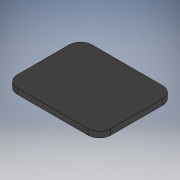
# Autodesk Inventor part: PODUSZKA PODSTAWY
Saved by Autodesk Inventor 2017 SP1 (Build 210196100, 196)
## iProperties
Created: 2020-12-24
Part Number: PODUSZKA PODSTAWY
Material: Kauczuk, silikon
Document SubType Name: Modeling
Designer: Napoleon
Mass: 0.902038 g
Surface Area: 10.8795 cm^2
Volume: 0.72163 cm^3
Density: 1.25 g/cm^3
Appearance: Kauczuk — czarny
Author: Napoleon
Autodesk Inventor part; units mm, degrees
ref_plane "YZ Plane" through (0, 0, 0) normal (1, 0, 0) x (0, 1, 0)
ref_plane "XZ Plane" through (0, 0, 0) normal (0, 1, 0) x (-1, 0, 0)
ref_plane "XY Plane" through (0, 0, 0) normal (0, 0, 1) x (1, 0, 0)
sketch "Szkic1" plane through (0, 0, 0) normal (0, 0, 1) x (1, 0, 0)
  line L0 (-9.375, -9.875) -> (9.375, -9.875)
  line L1 (12.375, -6.875) -> (12.375, 6.875)
  line L2 (9.375, 9.875) -> (-9.375, 9.875)
  line L3 (-12.375, 6.875) -> (-12.375, -6.875)
  arc A0 (-9.375, 9.875) -> (-12.375, 6.875) centre (-9.375, 6.875) ccw
  arc A1 (12.375, 6.875) -> (9.375, 9.875) centre (9.375, 6.875) ccw
  arc A2 (9.375, -9.875) -> (12.375, -6.875) centre (9.375, -6.875) ccw
  arc A3 (-12.375, -6.875) -> (-9.375, -9.875) centre (-9.375, -6.875) ccw
  point P0 (0, 0)
  point P1 (12.375, 9.875)
  point P2 (12.375, -9.875)
  point P3 (-12.375, 9.875)
  dimension "d0" = 24.75
  dimension "d1" = 19.75
  dimension "d2" = 3
  constraints: 8 end point, 8 point on circle, 8 tangent, 6 point on line, 4 centre point, 3 equal radius, 2 parallel, 1 horizontal, 1 perpendicular
  measures "d0" distance of point (-12.375, 9.875) point (12.375, 9.875)
  measures "d1" distance of point (12.375, 9.875) point (12.375, -9.875)
  measures "d2" radius of A0
extrude "Wyciągnięcie proste1" add sketch "Szkic1" along normal blind 1.5
